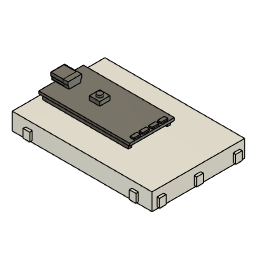
Simple MBed and Breadboard v6 (Autodesk Fusion 360 design; units mm, degrees)
Autodesk Fusion 360 part; units mm, degrees
sketch "Sketch1" plane through (0, 0, 0) normal (0, 1, 0) x (1, 0, 0)
  line L0 (0, 0) -> (83, 0) construction
  line L1 (83, 0) -> (83, -55.5) construction
  line L2 (83, -55.5) -> (0, -55.5) construction
  line L3 (0, -55.5) -> (0, 0) construction
  line L4 (0, 0) -> (81.5, 0)
  line L5 (0, 0) -> (0, -54)
  line L6 (81.5, 0) -> (81.5, -3)
  line L7 (81.5, -6.6) -> (83, -6.6) construction
  line L8 (83, -6.8) -> (81.5, -6.6)
  line L9 (83, -6.8) -> (83, -2.8)
  line L10 (83, -2.8) -> (81.5, -3)
  line L11 (81.5, 0) -> (81.5, -54) construction
  line L12 (81.5, -29.3) -> (82.9965, -29.3) construction
  line L13 (82.9965, -29.5) -> (81.5, -29.3)
  line L14 (82.9965, -29.5) -> (82.9965, -25.5)
  line L15 (82.9965, -25.5) -> (81.5, -25.7)
  line L16 (81.5, -25.7) -> (81.5, -6.6)
  line L17 (81.5, -29.3) -> (81.5, -25.7)
  line L18 (81.5, -6.6) -> (81.5, -3)
  line L19 (83, -25.7) -> (81.5, -25.7) construction
  line L20 (81.5, -54) -> (81.5, -51)
  line L21 (81.5, -51) -> (82.9965, -51) construction
  line L22 (83, -47.4) -> (81.5, -47.4) construction
  line L23 (81.5, -51) -> (81.5, -47.4)
  line L24 (82.9965, -51.2) -> (82.9965, -47.2)
  line L25 (82.9965, -47.2) -> (81.5, -47.4)
  line L26 (82.9965, -51.2) -> (81.5, -51)
  line L27 (81.5, -47.4) -> (81.5, -29.3)
  line L28 (81.5, -54) -> (0, -54)
  line L29 (0, -54) -> (8, -54) construction
  line L30 (81.5, -54) -> (73.5, -54) construction
  line L31 (69.9, -54) -> (69.9, -55.4965) construction
  line L32 (73.5, -55.5) -> (73.5, -54) construction
  line L33 (69.9, -54) -> (73.5, -54)
  line L34 (69.7, -55.4965) -> (73.7, -55.4965)
  line L35 (73.7, -55.4965) -> (73.5, -54)
  line L36 (69.7, -55.4965) -> (69.9, -54)
  line L37 (8, -54) -> (8, -55.4965) construction
  line L38 (11.6, -55.5) -> (11.6, -54) construction
  line L39 (8, -54) -> (11.6, -54)
  line L40 (7.8, -55.4965) -> (11.8, -55.4965)
  line L41 (11.8, -55.4965) -> (11.6, -54)
  line L42 (7.8, -55.4965) -> (8, -54)
  point P0 (83, -3)
  point P1 (83, -25.7)
  point P2 (83, -47.4)
  point P3 (73.5, -55.5)
  point P4 (11.6, -55.5)
  dimension "d1" = 83
  dimension "d2" = 55.5
  dimension "d3" = 81.5
  dimension "d4" = 54
  dimension "d10" = 3
  dimension "d11" = 0.2
  dimension "d12" = 4
  dimension "d13" = 0.2
  dimension "d14" = 54
  dimension "d16" = 0.2
  dimension "d17" = 4
  dimension "d18" = 0.2
  dimension "d94" = 3
  dimension "d95" = 0.2
  dimension "d96" = 4
  dimension "d97" = 0.2
  dimension "d99" = 8
  dimension "d100" = 8
  dimension "d101" = 0.2
  dimension "d102" = 4
  dimension "d103" = 0.2
  dimension "d104" = 0.2
  dimension "d105" = 4
  dimension "d106" = 0.2
  constraint horizontal L0
  constraint vertical L1
  constraint horizontal L2
  constraint vertical L3
  constraint coincident L0.start L3.end
  constraint perpendicular L3 L4
  constraint perpendicular L4 L5
  constraint perpendicular L0 L6
  constraint perpendicular L7 L9
  constraint vertical L11
  constraint perpendicular L12 L14
  constraint perpendicular L7 L16
  constraint perpendicular L12 L17
  constraint perpendicular L7 L18
  constraint horizontal L19
  constraint coincident P1 L19.start
  constraint parallel L11 L20
  constraint perpendicular L21 L24
  constraint perpendicular L21 L23
  constraint horizontal L22
  constraint coincident P2 L22.start
  constraint perpendicular L12 L27
  constraint perpendicular L3 L29
  constraint perpendicular L20 L30
  constraint perpendicular L31 L34
  constraint perpendicular L31 L33
  constraint coincident P3 L32.start
  constraint perpendicular L37 L40
  constraint perpendicular L37 L39
  constraint coincident P4 L38.start
  measures "d1" distance of L0.start L0.end
  measures "d2" distance of L0.start L2.end
  measures "d3" distance of L0.start L4.end
  measures "d4" distance of L0.start L5.end
  measures "d10" distance of L4.end L6.end
  measures "d11" distance of L8.start L7.end
  measures "d12" distance of L8.start L9.end
  measures "d13" distance of L9.end P0
  measures "d14" distance of L4.end L11.end
  measures "d16" distance of L13.start L12.end
  measures "d17" distance of L13.start L14.end
  measures "d18" distance of L14.end P1
  measures "d94" distance of L11.end L20.end
  measures "d95" distance of L24.start L21.end
  measures "d96" distance of L24.start L24.end
  measures "d97" distance of L24.end P2
  measures "d99" distance of L5.end L29.end
  measures "d100" distance of L11.end L30.end
  measures "d101" distance of L34.start L31.end
  measures "d102" distance of L34.start L34.end
  measures "d103" distance of L34.end P3
  measures "d104" distance of L40.start L37.end
  measures "d105" distance of L40.start L40.end
  measures "d106" distance of L40.end P4
extrude "Extrude1" add sketch "Sketch1" along normal blind 10 contours L4 L5 L6 L16 L17 L18 L20 L23 L27 L28 L33 L39 makes body 1
extrude "Extrude2" add sketch "Sketch1" along normal blind 6 contours L8 L9 L10 L18 | L28 L39 L40 L41 L42 | L13 L14 L15 L17 | L28 L33 L34 L35 L36 | L23 L24 L25 L26 bodies 1
extrude "Extrude3" cut sketch "Sketch1" along normal blind 1 contours L8 L9 L10 L18 | L28 L39 L40 L41 L42 | L13 L14 L15 L17 | L28 L33 L34 L35 L36 | L23 L24 L25 L26 bodies 1
sketch "Sketch2" plane through (0, 10, 0) normal (0, 1, 0) x (-1, 0, 0)
  line L0 (-81.5, 54) -> (-81.5, 0)
  line L1 (-81.5, 0) -> (0, 0)
  line L2 (0, 0) -> (0, 54)
  line L3 (0, 27) -> (-1.5, 27) construction
  line L4 (-1.5, 27) -> (-1.5, 40) construction
  line L5 (-1.5, 40) -> (-54.5, 40)
  line L6 (-54.5, 40) -> (-54.5, 14)
  line L7 (-54.5, 14) -> (-1.5, 14)
  line L8 (-1.5, 14) -> (-1.5, 40)
  line L9 (0, 27) -> (-24, 27) construction
  line L10 (-21, 30) -> (-27, 30)
  line L11 (-27, 30) -> (-27, 24)
  line L12 (-27, 24) -> (-21, 24)
  line L13 (-21, 24) -> (-21, 30)
  line L14 (-21, 30) -> (-27, 24) construction
  line L15 (-27, 30) -> (-21, 24) construction
  circle A0 centre (-24, 27) radius 1.6
  line L16 (0, 27) -> (-52.5, 27) construction
  line L17 (-52.7686, 27) -> (-52.7686, 19) construction
  line L18 (-51.7686, 21) -> (-53.7686, 21)
  line L19 (-53.7686, 21) -> (-53.7686, 17)
  line L20 (-53.7686, 17) -> (-51.7686, 17)
  line L21 (-51.7686, 17) -> (-51.7686, 21)
  line L22 (-51.7686, 21) -> (-53.7686, 17) construction
  line L23 (-53.7686, 21) -> (-51.7686, 17) construction
  line L24 (-52.7686, 27) -> (-52.7686, 24.25) construction
  line L25 (-53.7686, 22.25) -> (-51.7686, 22.25)
  line L26 (-51.7686, 22.25) -> (-51.7686, 26.25)
  line L27 (-51.7686, 26.25) -> (-53.7686, 26.25)
  line L28 (-53.7686, 26.25) -> (-53.7686, 22.25)
  line L29 (-53.7686, 22.25) -> (-51.7686, 26.25) construction
  line L30 (-51.7686, 22.25) -> (-53.7686, 26.25) construction
  line L31 (-52.7686, 27) -> (-52.7686, 29.75) construction
  line L32 (-52.7686, 27) -> (-52.7686, 35) construction
  line L33 (-53.7686, 27.75) -> (-51.7686, 27.75)
  line L34 (-51.7686, 27.75) -> (-51.7686, 31.75)
  line L35 (-51.7686, 31.75) -> (-53.7686, 31.75)
  line L36 (-53.7686, 31.75) -> (-53.7686, 27.75)
  line L37 (-53.7686, 27.75) -> (-51.7686, 31.75) construction
  line L38 (-51.7686, 27.75) -> (-53.7686, 31.75) construction
  line L39 (-53.7686, 33) -> (-51.7686, 33)
  line L40 (-51.7686, 33) -> (-51.7686, 37)
  line L41 (-51.7686, 37) -> (-53.7686, 37)
  line L42 (-53.7686, 37) -> (-53.7686, 33)
  line L43 (-53.7686, 33) -> (-51.7686, 37) construction
  line L44 (-51.7686, 33) -> (-53.7686, 37) construction
  line L45 (-1.5, 27) -> (-5.5, 27) construction
  line L46 (-1.5, 31) -> (-9.5, 31)
  line L47 (-9.5, 31) -> (-9.5, 23)
  line L48 (-9.5, 23) -> (-1.5, 23)
  line L49 (-1.5, 23) -> (-1.5, 31)
  line L50 (-1.5, 31) -> (-9.5, 23) construction
  line L51 (-9.5, 31) -> (-1.5, 23) construction
  line L52 (0, 54) -> (-81.5, 54)
  point P0 (-24, 27)
  point P1 (-52.7686, 19)
  point P2 (-52.7686, 24.25)
  point P3 (-52.7686, 29.75)
  point P4 (-52.7686, 35)
  point P5 (-5.5, 27)
  dimension "d40" = 1.5
  dimension "d41" = 13
  dimension "d42" = 53
  dimension "d43" = 26
  dimension "d44" = 24
  dimension "d45" = 6
  dimension "d46" = 6
  dimension "d47" = 3.2
  dimension "d48" = 52.5
  dimension "d49" = 8
  dimension "d50" = 2
  dimension "d51" = 4
  dimension "d52" = 2.75
  dimension "d53" = 2
  dimension "d54" = 4
  dimension "d55" = 2.75
  dimension "d56" = 8
  dimension "d57" = 2
  dimension "d58" = 4
  dimension "d59" = 2
  dimension "d60" = 4
  dimension "d61" = 4
  dimension "d62" = 8
  dimension "d63" = 8
  constraint midpoint L2 L3.start
  constraint perpendicular L2 L3
  constraint perpendicular L3 L4
  constraint horizontal L5
  constraint vertical L6
  constraint horizontal L7
  constraint vertical L8
  constraint perpendicular L2 L9
  constraint horizontal L10
  constraint perpendicular L10 L11
  constraint parallel L10 L12
  constraint parallel L11 L13
  constraint coincident L14 P0
  constraint coincident L15 P0
  constraint coincident P0 L9.end
  constraint perpendicular L2 L16
  constraint perpendicular L16 L17
  constraint horizontal L18
  constraint perpendicular L18 L19
  constraint parallel L18 L20
  constraint parallel L19 L21
  constraint coincident L22 P1
  constraint coincident L23 P1
  constraint coincident P1 L17.end
  constraint perpendicular L18 L24
  constraint horizontal L25
  constraint perpendicular L25 L26
  constraint parallel L25 L27
  constraint parallel L26 L28
  constraint coincident L29 P2
  constraint coincident L30 P2
  constraint coincident P2 L24.end
  constraint perpendicular L16 L31
  constraint perpendicular L16 L32
  constraint horizontal L33
  constraint perpendicular L33 L34
  constraint parallel L33 L35
  constraint parallel L34 L36
  constraint coincident L37 P3
  constraint coincident L38 P3
  constraint coincident P3 L31.end
  constraint horizontal L39
  constraint perpendicular L39 L40
  constraint parallel L39 L41
  constraint parallel L40 L42
  constraint coincident L43 P4
  constraint coincident L44 P4
  constraint coincident P4 L32.end
  constraint coincident L16 P5
  constraint horizontal L46
  constraint perpendicular L46 L47
  constraint parallel L46 L48
  constraint parallel L47 L49
  constraint coincident L50 P5
  constraint coincident L51 P5
  constraint coincident P5 L45.end
  measures "d40" distance of L3.start L3.end
  measures "d41" distance of L3.end L4.end
  measures "d42" distance of L4.end L5.end
  measures "d43" distance of L4.end L7.end
  measures "d44" distance of L3.start P0
  measures "d45" distance of L11.end L12.end
  measures "d46" distance of L10.end L11.end
  measures "d47" diameter of A0
  measures "d48" distance of L3.start L16.end
  measures "d49" distance of L17.start P1
  measures "d50" distance of L19.end L20.end
  measures "d51" distance of L18.end L19.end
  measures "d52" distance of L17.start P2
  measures "d53" distance of L26.end L27.end
  measures "d54" distance of L25.end L26.end
  measures "d55" distance of L17.start P3
  measures "d56" distance of L17.start P4
  measures "d57" distance of L34.end L35.end
  measures "d58" distance of L33.end L34.end
  measures "d59" distance of L40.end L41.end
  measures "d60" distance of L39.end L40.end
  measures "d61" distance of L3.end P5
  measures "d62" distance of L47.end L48.end
  measures "d63" distance of L46.end L47.end
extrude "Extrude4" add sketch "Sketch2" along normal blind 8 separate body contours L8 L46 L47 L48 L49 makes body 2
extrude "Extrude5" add sketch "Sketch2" along normal blind 7.6 contours A0 bodies 1
extrude "Extrude6" add sketch "Sketch2" along normal blind 6.3 contours L10 L11 L12 L13 bodies 1
extrude "Extrude7" add sketch "Sketch2" along normal blind 4.8 contours L18 L19 L20 L21 | L25 L26 L27 L28 | L33 L34 L35 L36 | L39 L40 L41 L42 bodies 1
extrude "Extrude8" add sketch "Sketch2" along normal blind 4 contours L5 L6 L7 L8 L46 L47 L48 bodies 1 2
extrude "Extrude9" add sketch "Sketch2" along normal blind 4 contours L5 L6 L7 L8 L46 L47 L48 bodies 1
sketch "Sketch3" plane through (1.5, 0, 0) normal (-1, 0, 0) x (0, 0, 1)
  line L0 (14, 10) -> (40, 10)
  line L1 (40, 10) -> (40, 14)
  line L2 (40, 14) -> (31, 14)
  line L3 (31, 14) -> (31, 18)
  line L4 (31, 18) -> (23, 18)
  line L5 (23, 18) -> (23, 14)
  line L6 (23, 14) -> (14, 14)
  line L7 (14, 14) -> (14, 10)
  line L8 (14, 14) -> (14, 12.5) construction
  line L9 (14, 12.5) -> (14.7, 12.5)
  line L10 (14.7, 12.5) -> (14.7, 10)
  line L11 (14.7, 10) -> (16.7, 10)
  line L12 (16.7, 10) -> (16.7, 12.5)
  line L13 (40, 12.5) -> (39.3, 12.5)
  line L14 (39.3, 12.5) -> (39.3, 10)
  line L15 (39.3, 10) -> (37.3, 10)
  line L16 (37.3, 10) -> (37.3, 12.5)
  line L17 (37.3, 12.5) -> (16.7, 12.5)
  line L18 (23, 16) -> (23.5657, 15.4343)
  line L19 (23, 16) -> (22.3, 16) construction
  line L20 (31, 16) -> (30.4343, 15.4343)
  line L21 (31, 16) -> (32.3, 16) construction
  line L22 (30.4343, 15.4343) -> (30.4343, 14)
  line L23 (30.4343, 14) -> (31, 14)
  line L24 (23.5657, 15.4343) -> (23.5657, 14)
  line L25 (23.5657, 14) -> (23, 14)
  line L26 (23.5657, 14) -> (30.4343, 14)
  line L27 (14.7, 12.5) -> (16.7, 12.5)
  line L28 (37.3, 12.5) -> (39.3, 12.5)
  line L29 (23, 16) -> (23, 18)
  line L30 (31, 16) -> (31, 18)
  line L31 (31, 18) -> (23, 18)
  line L32 (30.1843, 15.5379) -> (30.1843, 14.25)
  line L33 (23.8157, 14.25) -> (30.1843, 14.25)
  line L34 (23.8157, 15.5379) -> (23.8157, 14.25)
  line L35 (23.25, 16.1036) -> (23.8157, 15.5379)
  line L36 (23.25, 16.1036) -> (23.25, 17.75)
  line L37 (30.75, 17.75) -> (23.25, 17.75)
  line L38 (30.75, 16.1036) -> (30.75, 17.75)
  line L39 (30.75, 16.1036) -> (30.1843, 15.5379)
  line L40 (27, 14.25) -> (27, 17.75) construction
  line L41 (23, 16) -> (31, 16) construction
  line L42 (29.5, 17) -> (24.5, 17)
  line L43 (24.5, 17) -> (24.5, 15)
  line L44 (24.5, 15) -> (29.5, 15)
  line L45 (29.5, 15) -> (29.5, 17)
  line L46 (29.5, 17) -> (24.5, 15) construction
  line L47 (24.5, 17) -> (29.5, 15) construction
  line L48 (29.5, 16) -> (28.9226, 15)
  line L49 (29.5, 16) -> (29.6547, 16) construction
  line L50 (24.5, 16) -> (25.0774, 15)
  line L51 (24.5, 16) -> (22.3453, 16) construction
  point P0 (27, 16)
  dimension "d77" = 1.5
  dimension "d78" = 0.7
  dimension "d79" = 2
  dimension "d80" = 0.7
  dimension "d81" = 2
  dimension "d82" = 0.8
  dimension "d83" = 45
  dimension "d84" = 135
  dimension "d85" = 0.8
  dimension "d107" = -0.25
  dimension "d108" = 5
  dimension "d109" = 2
  dimension "d110" = 120
  dimension "d111" = 120
  constraint coincident L6.end L7.start
  constraint perpendicular L6 L8
  constraint perpendicular L7 L9
  constraint coincident L0 L10.end
  constraint perpendicular L0 L10
  constraint perpendicular L10 L11
  constraint perpendicular L9 L12
  constraint coincident L1 L13.start
  constraint perpendicular L1 L13
  constraint coincident L0 L14.end
  constraint perpendicular L0 L14
  constraint coincident L0 L15.end
  constraint perpendicular L13 L16
  constraint perpendicular L12 L17
  constraint horizontal L19
  constraint midpoint L5 L18.start
  constraint horizontal L21
  constraint midpoint L3 L20.start
  constraint perpendicular L2 L22
  constraint coincident L2.end L3.start
  constraint perpendicular L3 L23
  constraint perpendicular L23 L24
  constraint coincident L5.end L6.start
  constraint perpendicular L5 L25
  constraint perpendicular L12 L27
  constraint perpendicular L14 L28
  constraint coincident L4.end L5.start
  constraint coincident L3.end L4.start
  constraint midpoint L33 L40.start
  constraint midpoint L37 L40.end
  constraint horizontal L42
  constraint perpendicular L42 L43
  constraint parallel L42 L44
  constraint parallel L43 L45
  constraint coincident L46 P0
  constraint coincident L47 P0
  constraint midpoint L40 P0
  constraint horizontal L49
  constraint midpoint L45 L48.start
  constraint coincident L44 L48.end
  constraint horizontal L51
  constraint midpoint L43 L50.start
  constraint coincident L44 L50.end
  measures "d77" distance of L6.end L8.end
  measures "d78" distance of L8.end L9.end
  measures "d79" distance of L10.end L11.end
  measures "d80" distance of L13.start L13.end
  measures "d81" distance of L14.end L15.end
  measures "d82" distance of L18.start L18.end
  measures "d83" angle of L18 L19
  measures "d84" angle of L20 L21
  measures "d85" distance of L20.start L20.end
  measures "d108" distance of L43.end L44.end
  measures "d109" distance of L42.end L43.end
  measures "d110" angle of L48 L49
  measures "d111" angle of L50 L51
extrude "Extrude10" cut sketch "Sketch3" against normal blind 53 contours L0 L7 L9 L10 | L0 L12 L16 L17 | L0 L1 L13 L14 bodies 1
extrude "Extrude11" cut sketch "Sketch3" against normal blind 1.5 contours L0 L10 L11 L12 L27 | L0 L14 L15 L16 L28 bodies 1
extrude "Extrude14" cut sketch "Sketch3" against normal blind 5 contours L32 L33 L34 L35 L36 L37 L38 L39 | L44 L45 L48 | L43 L44 L50 bodies 1
extrude "Extrude15" cut sketch "Sketch3" against normal blind 8 contours L5 L18 L24 L25 | L3 L20 L22 L23 bodies 1
sketch "Sketch4" plane through (54.5, 0, 0) normal (1, 0, 0) x (0, 0, -1)
  line L0 (-16.7, 12.5) -> (-16.7, 10)
  line L1 (-16.7, 10) -> (-14.7, 10)
  line L2 (-14.7, 10) -> (-14.7, 12.5)
  line L3 (-14.7, 12.5) -> (-14, 12.5)
  line L4 (-14, 12.5) -> (-14, 14)
  line L5 (-14, 14) -> (-40, 14)
  line L6 (-40, 14) -> (-40, 12.5)
  line L7 (-40, 12.5) -> (-39.3, 12.5)
  line L8 (-39.3, 12.5) -> (-39.3, 10)
  line L9 (-39.3, 10) -> (-37.3, 10)
  line L10 (-37.3, 10) -> (-37.3, 12.5)
  line L11 (-37.3, 12.5) -> (-16.7, 12.5)
  line L12 (-16.7, 12.5) -> (-14.7, 12.5)
  line L13 (-39.3, 12.5) -> (-37.3, 12.5)
  constraint coincident L0.start L11.end
  constraint coincident L2.end L3.start
  constraint coincident L7.end L8.start
  constraint coincident L10.end L11.start
extrude "Extrude12" cut sketch "Sketch4" against normal blind 1.5 contours L0 L1 L2 L12 | L8 L9 L10 L13 bodies 1
extrude "Extrude13" add sketch "Sketch3" along normal blind 2 contours L3 L4 L5 L18 L20 L22 L24 L26 L29 L30 L31 bodies 1
split "Split1" by plane through (0, 10, 0) normal (0, 1, 0) bodies 1 makes body 3 at (27.6667, 14, 17.3333)
named bodies: "Breadboard", "MBed"
